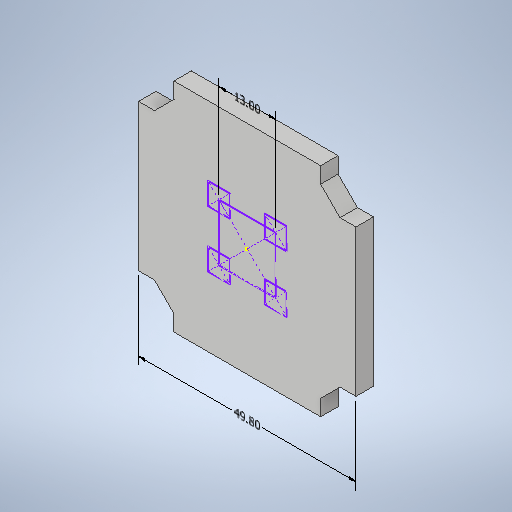
# Autodesk Inventor part: 样品池
Saved by Autodesk Inventor 2025.1 (Build 291241000, 241)
## iProperties
Created: 2024-08-29
Part Number: 样品池
Material: Generic
Document SubType Name: Sheet Metal
Designer: Administrator
Density: 1 g/cm^3
Sheet Metal Rule: 默认_mm
Appearance: Default
Author: Administrator
Autodesk Inventor part; units mm, degrees
ref_plane "YZ Plane" through (0, 0, 0) normal (1, 0, 0) x (0, 1, 0)
ref_plane "XZ Plane" through (0, 0, 0) normal (0, 1, 0) x (-1, 0, 0)
ref_plane "XY Plane" through (0, 0, 0) normal (0, 0, 1) x (1, 0, 0)
sketch "草图1" plane through (0, 0, 0) normal (0, 0, 1) x (1, 0, 0)
  line L0 (24.9, 0) -> (24.9, 16.8)
  line L1 (24.9, 16.8) -> (21.24, 16.8)
  line L2 (21.24, 16.8) -> (16.7994, 21.2406)
  line L3 (16.7994, 21.2406) -> (16.7994, 24.9006)
  line L4 (16.7994, 24.9006) -> (-0.0006, 24.9006)
  line L5 (-0.0006, 24.9006) -> (-16.8006, 24.9006)
  line L6 (-16.8006, 24.9006) -> (-16.8006, 21.2406)
  line L7 (-16.8006, 21.2406) -> (-21.2413, 16.8)
  line L8 (-21.2413, 16.8) -> (-24.9013, 16.8)
  line L9 (-24.9013, 16.8) -> (-24.9013, 0)
  line L10 (-24.9013, 0) -> (-24.9013, -16.8)
  line L11 (-24.9013, -16.8) -> (-21.2413, -16.8)
  line L12 (-21.2413, -16.8) -> (-16.8006, -21.2406)
  line L13 (-16.8006, -21.2406) -> (-16.8006, -24.9006)
  line L14 (-16.8006, -24.9006) -> (-0.0006, -24.9006)
  line L15 (-0.0006, -24.9006) -> (16.7994, -24.9006)
  line L16 (16.7994, -24.9006) -> (16.7994, -21.2406)
  line L17 (16.7994, -21.2406) -> (21.24, -16.8)
  line L18 (21.24, -16.8) -> (24.9, -16.8)
  line L19 (24.9, -16.8) -> (24.9, 0)
  point P0 (0, 0)
  constraints: 40 end point, 11 perpendicular, 2 collinear, 2 point on line, 2 vertical, 1 parallel
extrude "拉伸1" add sketch "草图1" along normal blind 4
sketch "草图2" plane through (0, 0, 4) normal (0, 0, 1) x (1, 0, 0)
  line L0 (-6.5, -6.5) -> (6.5, -6.5)
  line L1 (6.5, -6.5) -> (6.5, 6.5)
  line L2 (6.5, 6.5) -> (-6.5, 6.5)
  line L3 (-6.5, 6.5) -> (-6.5, -6.5)
  line L4 (-6.5, -6.5) -> (6.5, 6.5) construction
  line L5 (6.5, -6.5) -> (-6.5, 6.5) construction
  line L6 (-6.5, -6.5) -> (6.5, -6.5) construction
  line L7 (-6.5, 6.5) -> (-4.5, 6.5)
  line L8 (-9, 4) -> (-4, 4)
  line L9 (-4, 4) -> (-4, 9)
  line L10 (-4, 9) -> (-9, 9)
  line L11 (-9, 9) -> (-9, 4)
  line L12 (-9, 4) -> (-4, 9) construction
  line L13 (-4, 4) -> (-9, 9) construction
  line L14 (9, 4) -> (4, 4)
  line L15 (4, 4) -> (4, 9)
  line L16 (4, 9) -> (9, 9)
  line L17 (9, 9) -> (9, 4)
  line L18 (9, 4) -> (4, 9) construction
  line L19 (4, 4) -> (9, 9) construction
  line L20 (-9, -9) -> (-4, -9)
  line L21 (-4, -9) -> (-4, -4)
  line L22 (-4, -4) -> (-9, -4)
  line L23 (-9, -4) -> (-9, -9)
  line L24 (-9, -9) -> (-4, -4) construction
  line L25 (-4, -9) -> (-9, -4) construction
  line L26 (4, -4) -> (9, -4)
  line L27 (9, -4) -> (9, -9)
  line L28 (9, -9) -> (4, -9)
  line L29 (4, -9) -> (4, -4)
  line L30 (4, -4) -> (9, -9) construction
  line L31 (9, -4) -> (4, -9) construction
  point P0 (0, 0)
  constraints: 64 end point, 10 midpoint, 10 parallel, 5 perpendicular, 2 horizontal, 1 collinear, 1 point on line
equation "\"BendRadius\" = Thickness"
equation "\"BendReliefWidth\" = Thickness"
equation "\"BendReliefDepth\" = 0.5 * Thickness"
equation "\"CornerReliefSize\" = 4 * Thickness"
equation "\"MinimumRemnant\" = 2 * Thickness"
equation "\"TransitionRadius\" = BendRadius"
equation "\"JacobiRadiusSize\" = BendRadius"
equation "\"GapSize\" = Thickness"
equation "\"Thickness\" = 0.5"
